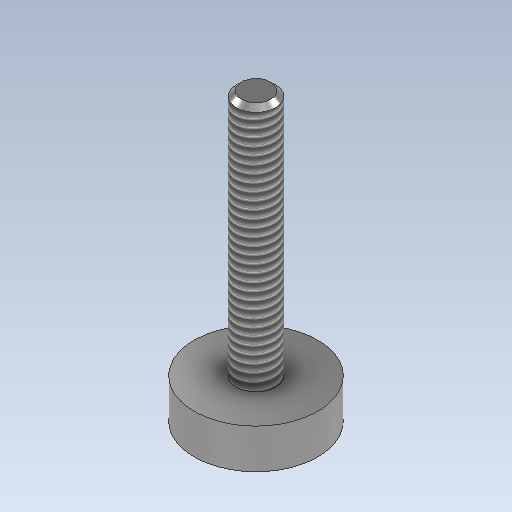
# Autodesk Inventor part: Pieza3
Saved by Autodesk Inventor 2020.3 (Build 243373000, 373)
## iProperties
Created: 2020-11-14
Part Number: Pieza3
Material: Acero inoxidable
Document SubType Name: Modeling
Designer: codig
Density: 8 g/cm^3
Appearance: Semipulido
Author: codig
Autodesk Inventor part; units mm, degrees
ref_plane "YZ Plane" through (0, 0, 0) normal (1, 0, 0) x (0, 1, 0)
ref_plane "XZ Plane" through (0, 0, 0) normal (0, 1, 0) x (-1, 0, 0)
ref_plane "XY Plane" through (0, 0, 0) normal (0, 0, 1) x (1, 0, 0)
sketch "Boceto1" plane through (0, 0, 0) normal (0, 1, 0) x (-1, 0, 0)
  circle A0 centre (0, 0) radius 12.5
  constraints: 1 centre point, 1 coincident
extrude "Extrusión1" add sketch "Boceto1" along normal blind 8
sketch "Boceto2" plane through (0, 8, 0) normal (0, 1, 0) x (1, 0, 0)
  circle A0 centre (0, 0) radius 4
  constraints: 1 centre point, 1 coincident
extrude "Extrusión2" add sketch "Boceto2" along normal blind 50
chamfer "Chaflán1" distance 1 angle 45 1 edges at (-4, 58, 0)
thread "Rosca1" size "3/8-16 UNC" class "1A" standard "ANSI Unified Screw Threads" full length
